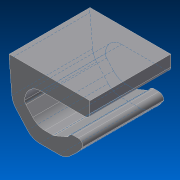
# Autodesk Inventor part: cable hook 4mm
Saved by Autodesk Inventor 2015 (Build 190159000, 159)
## iProperties
Created: 2017-03-21
Part Number: cable hook 4mm
Material: Generic
Document SubType Name: Modeling
Designer: ZigZagJoe
Density: 1 g/cm^3
Appearance: Default
Author: ZigZagJoe
Autodesk Inventor part; units mm, degrees
ref_plane "YZ Plane" through (0, 0, 0) normal (1, 0, 0) x (0, 1, 0)
ref_plane "XZ Plane" through (0, 0, 0) normal (0, 1, 0) x (-1, 0, 0)
ref_plane "XY Plane" through (0, 0, 0) normal (0, 0, 1) x (1, 0, 0)
sketch "Sketch1" plane through (0, 0, 0) normal (0, 1, 0) x (-1, 0, 0)
  line L0 (-4.2776, 1.7286) -> (5.7224, 1.7286)
  line L1 (5.7224, 1.7286) -> (5.7224, 1.1787)
  line L2 (5.7224, 1.1787) -> (5.3997, -2.5328)
  line L3 (4.9009, -3.6895) -> (3.4673, -5.2996)
  line L4 (1.9736, -5.9696) -> (-0.4363, -5.9696)
  line L5 (-1.7663, -5.4633) -> (-2.7917, -4.5503)
  line L6 (-2.8066, -3.0214) -> (-2.1946, -3.0214)
  line L7 (0.3597, -4.2714) -> (1.3256, -4.2714)
  line L8 (2.8192, -3.6014) -> (3.3548, -2.9999)
  line L9 (1.8097, -0.2714) -> (-3.6776, -0.2714)
  line L10 (-4.2776, 0.3286) -> (-4.2776, 1.7286)
  arc A0 (1.3256, -4.2714) -> (2.8192, -3.6014) centre (1.3256, -2.2714) ccw
  arc A1 (3.8097, -2.256) -> (1.8097, -0.2714) centre (1.8097, -2.2714) ccw
  arc A2 (1.9736, -5.9696) -> (3.4673, -5.2996) centre (1.9736, -3.9696) ccw
  arc A3 (-1.7663, -5.4633) -> (-0.4363, -5.9696) centre (-0.4363, -3.9696) ccw
  arc A4 (4.9009, -3.6895) -> (5.3997, -2.5328) centre (3.4072, -2.3595) ccw
  arc A5 (-2.8066, -3.0214) -> (-3.4028, -3.6891) centre (-2.8066, -3.6214) ccw
  arc A6 (-1.6666, -3.3365) -> (-2.1946, -3.0214) centre (-2.1946, -3.6214) ccw
  arc A7 (-4.2776, 0.3286) -> (-3.6776, -0.2714) centre (-3.6776, 0.3286) ccw
  line L11 (-2.7917, -4.5503) -> (-3.4028, -3.6891)
  line L12 (-1.3679, -3.606) -> (0.1303, -4.2258)
  arc A8 (-1.6666, -3.3365) -> (-1.3679, -3.606) centre (-1.1385, -3.0516) ccw
  line L13 (3.6578, -2.6596) -> (3.3548, -2.9999)
  arc A9 (3.6578, -2.6596) -> (3.8097, -2.256) centre (3.2097, -2.2606) ccw
  arc A10 (0.1303, -4.2258) -> (0.3597, -4.2714) centre (0.3597, -3.6714) ccw
  point P0 (0, 0)
  point P1 (3.7961, -2.5043)
  point P2 (-1.6055, -3.5077)
  dimension "d0" = 10
  dimension "d1" = 4
  dimension "d3" = 1.6
  dimension "d5" = 0.6
  dimension "d6" = 0.6
  dimension "d7" = 2.75
  dimension "d8" = 0.6
  dimension "d9" = 0.6
  dimension "d10" = 2
  constraints: 28 end point, 24 point on circle, 19 tangent, 11 centre point, 6 equal radius, 4 parallel, 4 perpendicular, 3 point on line, 1 horizontal
  measures "d0" distance of L0.start L0.end
  measures "d1" distance between parallel lines of L7 L9
  measures "d3" distance from line of L2 point (3.796, -2.504)
  measures "d5" radius of A5
  measures "d6" radius of A7
  measures "d7" distance between parallel lines of L6 L9
  measures "d8" radius of A8
  measures "d9" radius of A9
  measures "d10" distance between parallel lines of L9 L0
extrude "Extrusion1" add sketch "Sketch1" along normal blind 10
fillet "Fillet1" radius 5 1 edges at (2.7917, 5, -4.5503)
body "Solid1"
